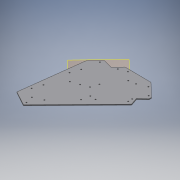
# Autodesk Inventor part: PlateRight
Saved by Autodesk Inventor 2018 (Build 220112000, 112)
## iProperties
Created: 2018-09-29
Part Number: PlateRight
Material: Generic
Document SubType Name: Modeling
Designer: eroldan
Density: 1 g/cm^3
Appearance: Default
Author: eroldan
Autodesk Inventor part; units mm, degrees
ref_plane "YZ Plane" through (0, 0, 0) normal (1, 0, 0) x (0, 1, 0)
ref_plane "XZ Plane" through (0, 0, 0) normal (0, 1, 0) x (-1, 0, 0)
ref_plane "XY Plane" through (0, 0, 0) normal (0, 0, 1) x (1, 0, 0)
ref_plane "Work Plane1" through (78.9702, 307.1183, 35) normal (0, 0, 1) x (0.6934154, 0.7205381, 0)
sketch "Sketch1" plane through (78.9702, 307.1183, 35) normal (0, 0, 1) x (0.6934154, 0.7205381, 0)
  line L0 (-245.8377, -151.2647) -> (102.2371, -154.4014)
  line L1 (102.2371, -154.4014) -> (118.2728, -123.5)
  line L2 (118.2728, -123.5) -> (166.8824, -126)
  line L3 (166.8824, -126) -> (166.8824, -34.5067)
  line L4 (166.8824, -34.5067) -> (85.4836, 52.2409)
  line L5 (-40.0118, 89.6338) -> (-265.4488, -79.16)
  line L6 (-265.4488, -79.16) -> (-245.8377, -151.2647)
  circle A0 centre (61.694, 42) radius 2.5 projected
  circle A1 centre (-56.306, 42) radius 2.5 projected
  circle A2 centre (94, 26.8002) radius 2.5 projected
  circle A3 centre (94, -23.1998) radius 2.5 projected
  circle A4 centre (118.7923, -42) radius 2.5 projected
  circle A5 centre (158.2014, -58.3927) radius 2.5 projected
  circle A6 centre (158.2014, -108.3927) radius 2.5 projected
  circle A7 centre (104.7371, -126) radius 2.5 projected
  circle A8 centre (-13.2629, -126) radius 2.5 projected
  circle A9 centre (-29.7986, -106.987) radius 2.5 projected
  circle A10 centre (-29.7986, -56.987) radius 2.5 projected
  circle A11 centre (0.7923, -42) radius 2.5 projected
  circle A12 centre (-61.3802, -42) radius 2.5 projected
  circle A13 centre (-94, -25.2342) radius 2.5 projected
  circle A14 centre (-94, 24.7658) radius 2.5 projected
  circle A15 centre (-217.7986, -110.5404) radius 2.5 projected
  circle A16 centre (-177.91, -126) radius 2.5 projected
  circle A17 centre (-217.7986, -60.5404) radius 2.5 projected
  circle A18 centre (-179.3802, -42) radius 2.5 projected
  circle A19 centre (-59.91, -126) radius 2.5 projected
  line L7 (85.4836, 52.2409) -> (40.182, 52.2409)
  line L8 (40.182, 52.2409) -> (19.661, 89.6338)
  line L9 (19.661, 89.6338) -> (-40.0118, 89.6338)
  circle A20 centre (4.6388, 81.3897) radius 2.5
  circle A21 centre (-235.861, -138.9507) radius 2.5
  circle A22 centre (91.5, -138.9507) radius 2.5
  point P0 (-276.0496, -156.0595)
  dimension "d5" = 5
  dimension "d6" = 5
  dimension "d7" = 5
  constraints: 20 end point, 3 centre point, 1 parallel
  measures "d5" diameter of A20
  measures "d6" diameter of A21
  measures "d7" diameter of A22
extrude "Extrusion1" add sketch "Sketch1" along normal blind 4
chamfer "Chamfer1" distance 8 angle 45 1 edges at (285.4768, 339.9931, 37)
body "Solid1"
